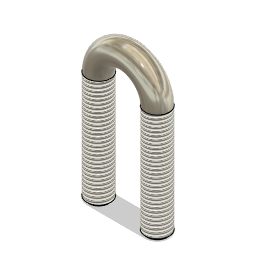
0.883.2423 - Etrier de 10x27x45 - IGTE 21400_17 Rep. 208 (Autodesk Fusion 360 design; units mm, degrees)
Autodesk Fusion 360 part; units mm, degrees
sketch "Sketch1" plane through (0, 0, 0) normal (0, 0, 1) x (1, 0, 0)
  line L0 (0, 0) -> (-12, 0) construction
  line L1 (0, 0) -> (12, 0) construction
  line L2 (-12, 0) -> (-12, -45)
  line L3 (12, 0) -> (12, -45)
  arc A0 (12, 0) -> (-12, 0) centre (0, 0) ccw
  dimension "d23" = 24
  dimension "d24" = 45
  dimension "d25" = 45
  constraint coincident L0.start L1.start
  constraint horizontal L0
  constraint parallel L0 L1
  measures "d23" diameter of A0
  measures "d24" distance of L0.end L2.end
  measures "d25" distance of L1.end L3.end
sketch "Sketch3" plane through (0, 0, 0) normal (0, 1, 0) x (1, 0, 0)
  circle A0 centre (12, 0) radius 5
  point P0 (12, 0)
  dimension "d26" = 10
  constraint coincident P0 A0.centre
  measures "d26" diameter of A0
sweep "Sweep1" add profiles "Sketch3" path "Sketch1" along L2 A0 L3 section 1
thread "Thread3" "ISO Metric profile 10.0 M10x1.5 6g" major diameter 9.85 minor diameter 8.141 pitch 1.5 angle 60 resizes the face on face at (-11.8753, -30, 4.9984)
thread "Thread4" "ISO Metric profile 10.0 M10x1.5 6g" major diameter 9.85 minor diameter 8.141 pitch 1.5 angle 60 resizes the face on face at (16.9189, -30, 0.2455)
chamfer "Chamfer2" distance 1 angle 45 1 edges at (-7.4083, -45, 1.781)
chamfer "Chamfer3" distance 1 angle 45 1 edges at (7.4083, -45, -1.781)
sketch "Sketch4 - construction positionnement" plane through (0, 0, 0) normal (0, 0, 1) x (1, 0, 0)
  circle A0 centre (0, 0) radius 6.075
  dimension "d29" = 12.15
  constraint coincident A0.centre origin
  measures "d29" diameter of A0
